receiverholder (Autodesk Fusion 360 design; units mm, degrees)
Autodesk Fusion 360 part; units mm, degrees
sketch "Sketch1" plane through (0, 0, 0) normal (0, 0, 1) x (1, 0, 0)
  line L0 (27, 25.5) -> (-27, 25.5)
  line L1 (-27, 25.5) -> (-27, -25.5)
  line L2 (-27, -25.5) -> (27, -25.5)
  line L3 (27, -25.5) -> (27, 25.5)
  line L4 (27, 25.5) -> (-27, -25.5) construction
  line L5 (-27, 25.5) -> (27, -25.5) construction
  line L6 (22.5, 12.5) -> (-22.5, -12.5) construction
  line L7 (-22.5, 12.5) -> (22.5, -12.5) construction
  line L8 (0, 0) -> (0, 17)
  line L9 (0, 0) -> (0, -17)
  circle A0 centre (0, 17) radius 2
  circle A1 centre (0, -17) radius 2
  dimension "d1" = 54
  dimension "d2" = 51
  dimension "d3" = 45
  dimension "d4" = 25
  dimension "d5" = 17
  dimension "d6" = 17
  dimension "d7" = 4
  dimension "d8" = 4
  constraint horizontal L0
  constraint perpendicular L0 L1
  constraint parallel L0 L2
  constraint parallel L1 L3
  constraint coincident L4 L8.start
  constraint coincident L5 L8.start
  constraint coincident L8.start L9.start
  constraint coincident L6 L8.start
  constraint coincident L7 L8.start
  constraint coincident L8.end A0.centre
  constraint coincident L9.end A1.centre
  measures "d1" distance of L1.end L2.end
  measures "d2" distance of L0.end L1.end
  measures "d3" distance of L6.end L7.end
  measures "d4" distance of L7.start L6.end
  measures "d5" distance of L8.start L8.end
  measures "d6" distance of L8.start L9.end
  measures "d7" diameter of A0
  measures "d8" diameter of A1
extrude "Extrude1" add sketch "Sketch1" along normal blind 2.4
ref_plane "WorkPlane1" through (0, 0, 2.4) normal (0, 0, 1) x (1, 0, 0)
sketch "Sketch3" plane through (0, 0, 2.4) normal (0, 0, 1) x (-1, 0, 0)
  circle A0 centre (0, 17) radius 2
  circle A1 centre (0, -17) radius 2
  line L0 (-27, 25.5) -> (-27, -25.5)
  line L1 (-27, -25.5) -> (27, -25.5)
  line L2 (27, -25.5) -> (27, 25.5)
  line L3 (27, 25.5) -> (-27, 25.5)
  line L4 (-22, 12.5) -> (22, 12.5)
  line L5 (22, 12.5) -> (22, -12.5)
  line L6 (22, -12.5) -> (-22, -12.5)
  line L7 (-22, -12.5) -> (-22, 12.5)
  line L8 (-22, 12.5) -> (22, -12.5) construction
  line L9 (22, 12.5) -> (-22, -12.5) construction
  line L10 (-23.8, 14.3) -> (23.8, 14.3)
  line L11 (23.8, 14.3) -> (23.8, -14.3)
  line L12 (23.8, -14.3) -> (-23.8, -14.3)
  line L13 (-23.8, -14.3) -> (-23.8, 14.3)
  line L14 (-23.8, -14.3) -> (23.8, -14.3)
  line L15 (23.8, -14.3) -> (23.8, -12.5)
  line L16 (22, -12.5) -> (-22, -12.5)
  line L17 (-23.8, -12.5) -> (-23.8, -14.3)
  line L18 (-23.8, 14.3) -> (23.8, 14.3)
  line L19 (23.8, 14.3) -> (23.8, 12.5)
  line L20 (-23.8, 12.5) -> (-23.8, 14.3)
  line L21 (17.4232, -14.3) -> (15.0232, -14.3)
  line L22 (15.0232, -14.3) -> (15.0232, -25.5)
  line L23 (15.0232, -25.5) -> (17.4232, -25.5)
  line L24 (17.4232, -25.5) -> (17.4232, -14.3)
  line L25 (0, -25.5) -> (0, 25.5)
  line L26 (27, 0) -> (-27, 0)
  line L27 (-17.4232, -14.3) -> (-15.0232, -14.3)
  line L28 (-15.0232, -14.3) -> (-15.0232, -25.5)
  line L29 (-15.0232, -25.5) -> (-17.4232, -25.5)
  line L30 (-17.4232, -25.5) -> (-17.4232, -14.3)
  line L31 (15.0232, 14.3) -> (15.0232, 25.5)
  line L32 (17.4232, 14.3) -> (15.0232, 14.3)
  line L33 (17.4232, 25.5) -> (17.4232, 14.3)
  line L34 (15.0232, 25.5) -> (17.4232, 25.5)
  line L35 (-17.4232, 14.3) -> (-15.0232, 14.3)
  line L36 (-17.4232, 25.5) -> (-17.4232, 14.3)
  line L37 (-15.0232, 14.3) -> (-15.0232, 25.5)
  line L38 (-15.0232, 25.5) -> (-17.4232, 25.5)
  dimension "d12" = 44
  dimension "d13" = 25
  dimension "d14" = -1.8
  dimension "d17" = 2.4
  constraint horizontal L4
  constraint perpendicular L4 L5
  constraint parallel L4 L6
  constraint parallel L5 L7
  constraint coincident L8 origin
  constraint coincident L9 origin
  constraint coincident L11 L15.end
  constraint coincident L11 L19.end
  constraint horizontal L14
  constraint vertical L15
  constraint horizontal L16
  constraint vertical L17
  constraint horizontal L18
  constraint vertical L19
  constraint vertical L20
  constraint horizontal L21
  constraint vertical L22
  constraint horizontal L23
  constraint vertical L24
  constraint coincident L12 L21.start
  constraint midpoint L1 L25.start
  constraint midpoint L3 L25.end
  constraint midpoint L2 L26.start
  constraint midpoint L0 L26.end
  constraint symmetric L21.start L25 L27.start
  constraint symmetric L21.end L25 L27.end
  constraint symmetric L22.end L25 L28.end
  constraint symmetric L23.end L25 L29.end
  constraint symmetric L21.start L26 L32.start
  constraint symmetric L21.end L26 L31.start
  constraint symmetric L22.end L26 L31.end
  constraint symmetric L23.end L26 L33.start
  constraint symmetric L26 L27.start L35.start
  constraint symmetric L26 L27.end L35.end
  constraint symmetric L26 L28.end L37.end
  constraint symmetric L26 L29.end L36.start
  measures "d12" distance of L5.end L6.end
  measures "d13" distance of L4.end L5.end
  measures "d17" distance of L21.start L21.end
extrude "Extrude2" add sketch "Sketch3" along normal blind 9 contours L4 L7 L10 L13 L18 L20 L25 L26 L35 | L4 L5 L10 L11 L18 L19 L25 L26 L32 | L6 L7 L12 L13 L14 L16 L17 L25 L26 L27 | L5 L6 L11 L12 L14 L15 L16 L21 L25 L26
extrude "Extrude3" add sketch "Sketch3" along normal blind 9 contours L3 L10 L18 L31 L32 L33 L34 | L3 L10 L18 L35 L36 L37 L38 | L1 L12 L14 L21 L22 L23 L24 | L1 L12 L14 L27 L28 L29 L30
sketch "Sketch4" plane through (0, 0, 0) normal (1, 0, 0) x (0, 1, 0)
  line L0 (0, 0) -> (0, 18.158)
  spline S0 degree 5 poles (22.0169, 12.3954) (22.115, 12.1372) (22.2812, 11.6469) (22.4403, 10.9895) (22.4713, 10.2698) (22.2114, 9.6276) (21.6709, 9.2232) (20.8914, 9.0138) (19.9508, 8.919) (18.9536, 8.8356) (18.0129, 8.6625) (17.2351, 8.3225) (16.7041, 7.7842) (16.4635, 7.0881) (16.526, 6.3227) (16.8851, 5.5971) (17.5246, 5.0142) (18.4293, 4.6453) (19.5853, 4.5365) (20.9805, 4.7143) (22.6053, 5.1912) (24.0832, 5.8146) (25.29, 6.4175) (26.138, 6.8793) (26.5729, 7.1252) knots 0 0 0 0 0 0 0.05 0.1 0.15 0.2 0.25 0.3 0.35 0.4 0.45 0.5 0.55 0.6 0.65 0.7 0.75 0.8 0.85 0.9 0.95 1 1 1 1 1 1
  line L1 (22.0169, 12.3954) -> (26.9177, 12.3954)
  line L2 (26.9177, 12.3954) -> (26.5729, 7.1252)
  line L3 (-22.0169, 12.3954) -> (-26.9177, 12.3954)
  spline S1 degree 5 poles (-22.0169, 12.3954) (-22.115, 12.1372) (-22.2812, 11.6469) (-22.4403, 10.9895) (-22.4713, 10.2698) (-22.2114, 9.6276) (-21.6709, 9.2232) (-20.8914, 9.0138) (-19.9508, 8.919) (-18.9536, 8.8356) (-18.0129, 8.6625) (-17.2351, 8.3225) (-16.7041, 7.7842) (-16.4635, 7.0881) (-16.526, 6.3227) (-16.8851, 5.5971) (-17.5246, 5.0142) (-18.4293, 4.6453) (-19.5853, 4.5365) (-20.9805, 4.7143) (-22.6053, 5.1912) (-24.0832, 5.8146) (-25.29, 6.4175) (-26.138, 6.8793) (-26.5729, 7.1252) knots 0 0 0 0 0 0 0.05 0.1 0.15 0.2 0.25 0.3 0.35 0.4 0.45 0.5 0.55 0.6 0.65 0.7 0.75 0.8 0.85 0.9 0.95 1 1 1 1 1 1
  line L4 (21.0791, 14.8624) -> (22.9546, 9.9284)
  line L5 (24.2002, 5.7836) -> (28.9455, 8.4668)
  line L6 (-21.0791, 14.8624) -> (-22.9546, 9.9284)
  line L7 (-24.2002, 5.7836) -> (-28.9455, 8.4668)
  line L8 (-26.9177, 12.3954) -> (-26.5729, 7.1252)
  circle A0 centre (-7.6182, 6.6) radius 2
  line L9 (14.3, 2.4) -> (-14.3, 2.4)
  line L10 (-25.5, 2.4) -> (-14.3, 2.4)
  line L11 (25.5, 2.4) -> (14.3, 2.4)
  circle A1 centre (7.6182, 6.6) radius 2
  line L12 (-14.3, 11.4) -> (14.3, 11.4)
  line L13 (-11.5361, 2.4) -> (-11.5361, 14.44)
  line L14 (11.5361, 2.4) -> (11.5361, 14.44)
  line L15 (-11.5361, 11.4) -> (11.5361, 11.4)
  line L16 (11.5361, 11.4) -> (11.5361, 5.4)
  line L17 (11.5361, 5.4) -> (-11.5361, 5.4)
  line L18 (-11.5361, 5.4) -> (-11.5361, 11.4)
  point P0 (21.4258, 9.1939)
  point P1 (17.2392, 8.2334)
  point P2 (16.9437, 5.6476)
  point P3 (-21.4258, 9.1939)
  point P4 (-17.2392, 8.2334)
  point P5 (-16.9437, 5.6476)
  dimension "d23" = 4
  dimension "d24" = 4.2
  dimension "d25" = 3
  constraint coincident L0.start origin
  constraint vertical L0
  constraint horizontal L1
  constraint midpoint S0.start L4
  constraint midpoint S0.end L5
  constraint symmetric L0 S0.start L3.start
  constraint symmetric L0 P0 P3
  constraint symmetric L0 P1 P4
  constraint symmetric L0 P2 P5
  constraint symmetric L0 S0.end S1.end
  constraint symmetric L0 L1.end L3.end
  constraint symmetric L0 L4.start L6.start
  constraint symmetric L0 L4.end L6.end
  constraint symmetric L0 L5.start L7.start
  constraint symmetric L0 L5.end L7.end
  constraint symmetric L0 A0 A1
  constraint coincident L9 L13.start
  constraint perpendicular L12 L13
  constraint symmetric L0 L13.start L14.start
  constraint symmetric L0 L13.end L14.end
  constraint horizontal L15
  constraint vertical L16
  constraint horizontal L17
  constraint vertical L18
  constraint coincident L14 L16.end
  constraint coincident L13 L15.start
  constraint coincident L12 L15.start
  measures "d23" diameter of A0
  measures "d24" distance of A0.centre L9
  measures "d25" distance of L9 L17
extrude "Extrude4" cut sketch "Sketch4" along normal mid plane 41 contours S0 L1 L2
extrude "Extrude5" cut sketch "Sketch4" along normal through all and the other way through all contours L3 S1 L8
extrude "Extrude6" cut sketch "Sketch4" against normal through all contours A1 L17 | A0 L17 picked at (8.2114, 6.2331) picked at (-7.1462, 7.2911)
extrude "Extrude7" cut sketch "Sketch4" along normal through all contours L0 A0 L12 L13 L15 L17 L18 | L0 A1 L12 L14 L15 L16 L17 | A1 L17 | A0 L17 picked at (8.2114, 6.2331) picked at (-7.1462, 7.2911)
fillet "Fillet1" radius 3.5 4 edges at (-27, -25.5, 1.2) (27, -25.5, 1.2) (27, 25.5, 1.2) (-27, 25.5, 1.2)
fillet "Fillet2" radius 1 4 edges at (-16.2232, -25.5, 6.5412) (16.2232, -25.5, 6.5412) (-16.2232, 25.5, 6.5412) (16.2232, 25.5, 6.5412)
fillet "Fillet3" radius 1 4 edges at (-16.2232, 22.3236, 11.4) (16.2232, 22.3236, 11.4) (-16.2232, -22.3236, 11.4) (16.2232, -22.3236, 11.4)
chamfer "Chamfer1" distance 1.2 angle 45 8 edges at (-15.0232, 14.3, 6.9) (15.0232, 14.3, 6.9) (-17.4232, 14.3, 6.9) (17.4232, 14.3, 6.9) (17.4232, -14.3, 6.9) (15.0232, -14.3, 6.9) (-15.0232, -14.3, 6.9) (-17.4232, -14.3, 6.9)
